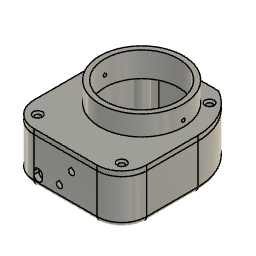
Microscope illuminator (Autodesk Fusion 360 design; units mm, degrees)
Autodesk Fusion 360 part; units mm, degrees
sketch "Sketch1" plane through (0, 0, 0) normal (0, 0, 1) x (1, 0, 0)
  circle A0 centre (0, 0) radius 25.2
  line L0 (-34, 0) -> (0, 0) construction
  line L1 (34, 0) -> (0, 0) construction
  line L2 (-10, 21) -> (10, 21) construction
  line L3 (10, 21) -> (10, -39) construction
  line L4 (10, -39) -> (-10, -39) construction
  line L5 (-10, -39) -> (-10, 21) construction
  line L6 (0, -39) -> (0, 0) construction
  circle A1 centre (0, 0) radius 5 construction
  arc A2 (34, 0) -> (-34, 0) centre (0, 0) ccw
  line L7 (-34, 0) -> (-34, -46)
  line L8 (34, 0) -> (34, -46)
  line L9 (34, -46) -> (-34, -46)
  circle A3 centre (0, 0) radius 22.2
  line L10 (16.9041, 29.5) -> (-16.9041, 29.5)
  line L11 (0, 0) -> (0, 34) construction
  dimension "d3" = 50.4
  dimension "d4" = 68
  dimension "d5" = 60
  dimension "d6" = 20
  dimension "d7" = 39
  dimension "d8" = 10
  dimension "d9" = 3
  dimension "d11" = 46
  dimension "d65" = 4.5
  constraint concentric A0 A2
  constraint coincident A0.centre L0.end
  constraint horizontal L0
  constraint horizontal L2
  constraint vertical L3
  constraint horizontal L4
  constraint vertical L5
  constraint midpoint L4 L6.start
  constraint perpendicular L4 L6
  constraint tangent A2 L7
  constraint tangent A2 L8
  constraint perpendicular L1 L8
  constraint horizontal L9
  constraint concentric A2 A3
  constraint perpendicular L8 L9
  constraint coincident A2 L10.start
  constraint coincident A2 L10.end
  constraint parallel L1 L10
  constraint midpoint A2 L11.end
  measures "d3" diameter of A0
  measures "d4" diameter of A2
  measures "d5" distance of L2.start L4.end
  measures "d6" distance of L2.start L2.end
  measures "d7" distance of L6.start A0.centre
  measures "d8" diameter of A1
  measures "d9" distance of A0 A3
  measures "d11" distance of L0.start L7.end
  measures "d65" distance of L10 L11.end
extrude "Extrude1" add sketch "Sketch1" along normal blind 15 contours A0 makes body 1
extrude "Extrude2" add sketch "Sketch1" along normal blind 3 contours A2 L7 L8 L9 L10 bodies 1
sketch "Sketch Mounting Ring Holes" plane through (0, 0, 0) normal (1, 0, 0) x (0, 1, 0)
  line L0 (0, 15) -> (0, 3) construction
  circle A0 centre (0, 6.5) radius 1
  point P0 (0, 3)
  point P1 (0, 15)
  dimension "d16" = 2
  dimension "d130" = 3.5
  constraint coincident P1 L0.start
  constraint coincident P0 L0.end
  measures "d16" diameter of A0
  measures "d130" distance of P0 A0.centre
extrude "Extrude3" cut sketch "Sketch Mounting Ring Holes" along normal through all and the other way through all bodies 1
fillet "Fillet1" radius 15 2 edges at (-34, -46, 1.5) (34, -46, 1.5) on bodies 1
sketch "Sketch Body Profile" plane through (0, 0, 0) normal (0, 0, 1) x (1, 0, 0)
  arc A0 (19, -46) -> (34, -31) centre (19, -31) ccw
  line L0 (19, -46) -> (-19, -46)
  arc A1 (-34, -31) -> (-19, -46) centre (-19, -31) ccw
  line L1 (-34, -31) -> (-34, 0)
  arc A2 (-16.9041, 29.5) -> (-34, 0) centre (0, 0) ccw
  line L2 (34, 0) -> (34, -31)
  circle A3 centre (0, 0) radius 22.2
  line L3 (-16.9041, 29.5) -> (16.9041, 29.5)
  arc A4 (34, 0) -> (16.9041, 29.5) centre (0, 0) ccw
extrude "Extrude4" add sketch "Sketch Body Profile" against normal blind 27 separate body contours A0 L0 A1 L1 A2 L2 L3 A4 | A3 makes body 2
fillet "Fillet2" radius 3 8 edges at (29.6066, -41.6066, -27) (0, -46, -27) (-29.6066, -41.6066, -27) (-34, -15.5, -27) (-29.4172, 17.0479, -27) (34, -15.5, -27) (29.4172, 17.0479, -27) (0, 29.5, -27) on bodies 2
shell "Shell1" thickness 3 removed faces 1 at (6.3333, -15.3333, 0) on bodies 2
sketch "Sketch Lamp Base Mounting Bosses" plane through (0, -43, 0) normal (0, -1, 0) x (1, 0, 0)
  line L0 (-19, -27) -> (19, -27)
  line L1 (19, -27) -> (19, 0)
  line L2 (19, 0) -> (-19, 0)
  line L3 (-19, 0) -> (-19, -27)
  line L4 (0, 0) -> (0, -27) construction
  circle A0 centre (0, -13.5) radius 6.375 construction
  line L5 (0, -13.5) -> (3.6565, -8.2779) construction
  circle A1 centre (3.6565, -8.2779) radius 1.75
  line L6 (3.6565, -8.2779) -> (-3.6565, -18.7221) construction
  circle A2 centre (-3.6565, -18.7221) radius 1.75
  circle A3 centre (-3.6565, -18.7221) radius 3.75
  circle A4 centre (3.6565, -8.2779) radius 3.75
  line L7 (3.6565, -8.2779) -> (3.6565, -6.5279) construction
  line L8 (3.6565, -6.5279) -> (3.6565, -6.0279) construction
  line L9 (3.6565, -6.0279) -> (4.7565, -6.9168)
  line L10 (3.6565, -6.0279) -> (2.5566, -6.9168)
  line L11 (-3.6565, -18.7221) -> (-3.6565, -16.9721) construction
  line L12 (-3.6565, -16.9721) -> (-3.6565, -16.4721) construction
  line L13 (-3.6565, -16.4721) -> (-2.5566, -17.361)
  line L14 (-3.6565, -16.4721) -> (-4.7565, -17.361)
  line L15 (3.1565, -11.9944) -> (4.1565, -11.9944)
  line L16 (-4.1565, -22.4386) -> (-3.1565, -22.4386)
  line L17 (19, -24) -> (-19, -24)
  line L18 (-19, -24) -> (-19, 0)
  line L19 (-19, 0) -> (19, 0)
  line L20 (19, 0) -> (19, -24)
  dimension "d26" = 35
  dimension "d27" = 3.5
  dimension "d28" = 3.5
  dimension "d31" = 2
  dimension "d32" = 2
  dimension "d66" = 12.75
  dimension "d67" = 0.5
  dimension "d68" = 0.5
  dimension "d69" = 1
  dimension "d70" = 1
  constraint coincident L4.start origin
  constraint midpoint L0 L4.end
  constraint midpoint L4 A0.centre
  constraint coincident A0.centre L5.start
  constraint coincident A0 L5.end
  constraint coincident L5.end A1.centre
  constraint coincident A0 L6.end
  constraint parallel L5 L6
  constraint coincident L6.end A2.centre
  constraint concentric A2 A3
  constraint coincident A1 L7.end
  constraint vertical L7
  constraint parallel L7 L8
  constraint coincident A1 L9.end
  constraint tangent A1 L9
  constraint coincident A1 L10.end
  constraint tangent A1 L10
  constraint coincident A2 L11.end
  constraint vertical L11
  constraint parallel L11 L12
  constraint coincident A2 L13.end
  constraint tangent A2 L13
  constraint coincident A2 L14.end
  constraint tangent A2 L14
  constraint coincident A4 L15.start
  constraint coincident A4 L15.end
  constraint horizontal L15
  constraint coincident A3 L16.start
  constraint coincident A3 L16.end
  constraint horizontal L16
  measures "d26" angle of L4 L5
  measures "d27" diameter of A1
  measures "d28" diameter of A2
  measures "d31" distance of A1 A4
  measures "d32" distance of A2 A3
  measures "d66" distance of L5.end L6.end
  measures "d67" distance of L7.end L8.end
  measures "d68" distance of L11.end L12.end
  measures "d69" distance of L15.start L15.end
  measures "d70" horizontal distance of L16.start L16.end
extrude "Extrude5" add sketch "Sketch Lamp Base Mounting Bosses" against normal blind 3 contours A3 L16 | A4 L15 picked at (-2.8156, -16.3619) picked at (4.4975, -5.9177) bodies 2
extrude "Extrude6" cut sketch "Sketch Lamp Base Mounting Bosses" along normal up to surface (3 mm away) contours A1 | A1 L9 L10 | A2 | A2 L13 L14 bodies 2
box "BoxPrimitive1" add length 3 width 1 height 3 placed x (0, -1, 0) y (-1, 0, 0) z (0, 0, -1) at (4.1565, -40, -11.9944) bodies 2
box "BoxPrimitive2" add length 3 width 1 height 3 placed x (0, -1, 0) y (-1, 0, 0) z (0, 0, -1) at (-3.1565, -40, -22.4386) bodies 2
chamfer "Chamfer2" distance 3 angle 45 1 edges at (3.6565, -40, -14.9944) on bodies 2
sketch "Sketch Screw Bosses in Base" plane through (0, 0, -24) normal (0, 0, 1) x (-1, 0, 0)
  line L0 (-20, 0) -> (-2.5, 0)
  line L1 (0, 0) -> (0, 23.7257) construction
  line L2 (0, 0) -> (-24.0416, -24.0416) construction
  circle A0 centre (-20.5061, -20.5061) radius 4
  arc A1 (16.9041, -29.5) -> (34, 0) centre (0, 0) ccw
  line L3 (-22.5355, 34.5355) -> (-29.6066, 41.6066) construction
  line L4 (-19, 43) -> (19, 43)
  arc A2 (-19, 46) -> (-34, 31) centre (-19, 31) ccw
  circle A3 centre (-25.364, 37.364) radius 4
  circle A4 centre (-20.5061, -20.5061) radius 1.15
  circle A5 centre (-25.364, 37.364) radius 1.15
  circle A6 centre (20.5061, -20.5061) radius 4
  circle A7 centre (20.5061, -20.5061) radius 1.15
  circle A8 centre (25.364, 37.364) radius 4
  circle A9 centre (25.364, 37.364) radius 1.15
  line L5 (31, 0) -> (31, 31)
  arc A10 (31, 31) -> (19, 43) centre (19, 31) ccw
  line L6 (3.1565, 43) -> (-19, 43)
  arc A11 (-19, 43) -> (-31, 31) centre (-19, 31) ccw
  line L7 (-31, 31) -> (-31, 0)
  arc A12 (16.0857, -26.5) -> (31, 0) centre (0, 0) ccw
  arc A13 (-31, 0) -> (-16.0857, -26.5) centre (0, 0) ccw
  line L8 (-16.0857, -26.5) -> (16.0857, -26.5)
  line L9 (4.1565, 43) -> (4.1565, 40)
  line L10 (4.1565, 40) -> (3.1565, 40)
  line L11 (3.1565, 40) -> (3.1565, 43)
  line L12 (19, 43) -> (4.1565, 43)
  dimension "d48" = 45
  dimension "d49" = 8
  dimension "d50" = 5
  dimension "d51" = 45
  dimension "d52" = 8
  dimension "d53" = 6
  dimension "d54" = 2.3
  dimension "d56" = 2.3
  constraint perpendicular L0 L1
  constraint coincident L1.start L2.start
  constraint coincident L2 A0.centre
  constraint coincident L2.end A1
  constraint midpoint L3.end A2
  constraint coincident L3 A3.centre
  constraint concentric A0 A4
  constraint concentric A3 A5
  constraint symmetric L1 A0 A6
  constraint symmetric L1 A3 A8
  constraint symmetric L1 A4 A7
  constraint symmetric L1 A5 A9
  measures "d48" angle of L0 L2
  measures "d49" diameter of A0
  measures "d50" distance of L2.end A0.centre
  measures "d51" angle of L3 L4
  measures "d52" diameter of A3
  measures "d53" distance of L3.end A3.centre
  measures "d54" diameter of A4
  measures "d56" diameter of A5
extrude "Extrude9" add sketch "Sketch Screw Bosses in Base" along normal up to surface (24 mm away) contours A0 A13 | A0 A13 | A3 A11 | A3 A11 | A6 A12 | A6 A12 | A8 A10 | A8 A10 bodies 2
sketch "Sketch Lid Mounting Hole Location" plane through (0, 0, 3) normal (0, 0, 1) x (-1, 0, 0)
  arc A0 (-19, 46) -> (-34, 31) centre (-19, 31) ccw
  line L0 (-34, 31) -> (-34, 0)
  arc A1 (-34, 0) -> (-16.9041, -29.5) centre (0, 0) ccw
  line L1 (34, 0) -> (34, 31)
  arc A2 (34, 31) -> (19, 46) centre (19, 31) ccw
  line L2 (19, 46) -> (-19, 46)
  circle A3 centre (0, 0) radius 25.2
  line L3 (-16.9041, -29.5) -> (16.9041, -29.5)
  arc A4 (16.9041, -29.5) -> (34, 0) centre (0, 0) ccw
  point P0 (25.364, 37.364)
  point P1 (-25.364, 37.364)
  point P2 (20.5061, -20.5061)
  point P3 (-20.5061, -20.5061)
hole "Hole1" at (-25.364, -37.364, 3) at (25.364, -37.364, 3) at (-20.5061, 20.5061, 3) at (20.5061, 20.5061, 3) direction (0, 0, -1) diameter 3.3 depth 4 tip angle 118 countersink diameter 5.5 countersink angle 90 bodies 1
sketch "Sketch Zip Tie Loop" plane through (-31, 0, 0) normal (1, 0, 0) x (0, 1, 0)
  line L0 (0, -24) -> (0, 0)
  line L1 (0, 0) -> (-31, 0)
  line L2 (-31, 0) -> (-31, -24)
  line L3 (-31, -24) -> (0, -24)
  line L4 (-43, -22.4386) -> (-43, -24)
  line L5 (-43, -24) -> (-43, 0)
  line L6 (-43, 0) -> (-43, -24)
  line L7 (-43, -24) -> (-43, -22.4386)
  line L8 (-43, -14.9721) -> (-43, -22.4386)
  line L9 (-43, -14.9944) -> (-43, -11.9944)
  line L10 (-43, -4.5279) -> (-43, -11.9944)
  line L11 (-43, -11.9944) -> (-43, -14.9944)
  line L12 (-24, -24) -> (-24, -16)
  line L13 (-24, -16) -> (-14, -16)
  line L14 (-14, -16) -> (-14, -24)
  line L15 (-43, 0) -> (-43, -24)
  line L16 (-24, -24) -> (-14, -24)
  point P0 (-43, -24)
  point P1 (-43, -24)
  point P2 (-43, -24)
  dimension "d111" = 8
  dimension "d112" = 10
  dimension "d114" = 19
  constraint coincident L3 L12.start
  constraint perpendicular L3 L12
  constraint perpendicular L12 L13
  constraint coincident L3 L14.end
  constraint perpendicular L3 L14
  measures "d111" distance of L12.start L12.end
  measures "d112" distance of L12.end L13.end
  measures "d114" distance of L9.start L12
extrude "Extrude14" add sketch "Sketch Zip Tie Loop" along normal blind 6 contours L3 L12 L13 L14 L16 bodies 2
sketch "Sketch Zip Tie Loop top" plane through (0, 0, -16) normal (0, 0, 1) x (-1, 0, 0)
  line L0 (31, 14) -> (31, 24)
  line L1 (31, 24) -> (25, 24)
  line L2 (25, 24) -> (25, 14)
  line L3 (25, 14) -> (31, 14)
  line L4 (25, 19) -> (31, 19) construction
  line L5 (31, 21.5) -> (27, 21.5)
  line L6 (31, 16.5) -> (27, 16.5)
  line L7 (27, 21.5) -> (27, 16.5)
  line L8 (31, 24) -> (31, 14)
  dimension "d118" = 5
  dimension "d119" = 4
  constraint midpoint L2 L4.start
  constraint midpoint L0 L4.end
  constraint coincident L0 L5.start
  constraint perpendicular L0 L5
  constraint symmetric L4 L5.start L6.start
  constraint symmetric L4 L5.end L6.end
  measures "d118" distance of L5.end L6.end
  measures "d119" distance of L7 L8
extrude "Extrude15" cut sketch "Sketch Zip Tie Loop top" against normal up to surface (8 mm away) contours L0 L5 L6 L7 L8 bodies 2
sketch "Sketch19" plane through (-25, 0, 0) normal (1, 0, 0) x (0, 1, 0)
  line L0 (-24, -16) -> (-24, -24)
  line L1 (-24, -24) -> (-14, -24)
  line L2 (-14, -24) -> (-14, -16)
  line L3 (-14, -16) -> (-24, -16)
  line L4 (-24, -24) -> (-24, -16)
  line L5 (-24, -16) -> (-21.5, -16)
  line L6 (-21.5, -16) -> (-21.5, -24)
  line L7 (-21.5, -24) -> (-16.5, -24)
  line L8 (-16.5, -24) -> (-16.5, -16)
  line L9 (-16.5, -16) -> (-14, -16)
  line L10 (-14, -16) -> (-14, -24)
  line L11 (-14, -24) -> (0, -24)
  line L12 (0, -24) -> (0, 0)
  line L13 (0, 0) -> (-31, 0)
  line L14 (-31, 0) -> (-31, -24)
  line L15 (-31, -24) -> (-24, -24)
  line L16 (-16.5, -19) -> (-21.5, -19)
  line L17 (-21.5, -19) -> (-21.5, -24)
  line L18 (-16.5, -24) -> (-16.5, -19)
  dimension "d124" = 3
  constraint coincident L8 L16.start
  constraint coincident L6 L16.end
  constraint perpendicular L6 L16
  constraint coincident L6.end L7.start
  constraint perpendicular L7 L17
  constraint coincident L7.end L8.start
  constraint perpendicular L7 L18
  measures "d124" distance of L3 L16
extrude "Extrude16" cut sketch "Sketch19" against normal up to surface (6 mm away) contours L1 L6 L7 L8 L16 L17 L18 bodies 2
fillet "Fillet3" radius 1 1 edges at (-31, -19, -24) on bodies 2
chamfer "Chamfer6" distance 1 angle 45 2 edges at (-26, -21.5, -19) (-26, -16.5, -19) on bodies 2
sketch "Sketch Lamp Cord Hole" plane through (0, -43, 0) normal (0, -1, 0) x (1, 0, 0)
  line L0 (-4.1565, -22.4386) -> (-4.1565, -24)
  line L1 (-4.1565, -24) -> (-19, -24)
  line L2 (-19, -24) -> (-19, 0)
  line L3 (-19, 0) -> (19, 0)
  line L4 (19, 0) -> (19, -24)
  line L5 (19, -24) -> (-3.1565, -24)
  line L6 (-3.1565, -24) -> (-3.1565, -22.4386)
  arc A0 (-3.1565, -22.4386) -> (-4.1565, -22.4386) centre (-3.6565, -18.7221) ccw
  line L7 (4.1565, -14.9944) -> (4.1565, -11.9944)
  arc A1 (4.1565, -11.9944) -> (3.1565, -11.9944) centre (3.6565, -8.2779) ccw
  line L8 (3.1565, -11.9944) -> (3.1565, -14.9944)
  line L9 (3.1565, -14.9944) -> (4.1565, -14.9944)
  line L10 (-19, -19) -> (-19, -21)
  arc A2 (-19, -21) -> (-14, -21) centre (-16.5, -21) ccw
  line L11 (-14, -21) -> (-14, -19)
  arc A3 (-14, -19) -> (-19, -19) centre (-16.5, -19) ccw
  line L12 (-16.5, -19) -> (-16.5, -21) construction
  line L13 (-16.5, -19) -> (-16.5, -16.5) construction
  line L14 (-16.5, -21) -> (-16.5, -23.5) construction
  line L15 (-16.5, -20) -> (-19, -12) construction
  line L16 (19, -24) -> (-19, -24) construction
  dimension "d97" = 5
  dimension "d98" = 7
  dimension "d99" = 2.5
  dimension "d100" = 0.5
  constraint tangent L10 A2
  constraint tangent A2 L11
  constraint parallel L10 L11
  constraint tangent L11 A3
  constraint tangent L10 A3
  constraint perpendicular L3 L12
  constraint coincident A3.centre L12.start
  constraint midpoint A3 L13.end
  constraint coincident A2.centre L12.end
  constraint midpoint A2 L14.end
  constraint midpoint L12 L15.start
  constraint midpoint L2 L15.end
  measures "d97" distance of L10 L11
  measures "d98" distance of L13.end L14.end
  measures "d99" horizontal distance of L15.start L15.end
  measures "d100" distance of L14.end L16
extrude "Extrude12" cut sketch "Sketch Lamp Cord Hole" along normal up to surface (3 mm away) contours L2 L10 A2 L11 A3 bodies 2
sketch "Sketch LED Only text" plane through (0, 0, -24) normal (0, 0, 1) x (-1, 0, 0)
  line L0 (31, 24) -> (31, 31)
  arc A0 (31, 31) -> (29.353, 37.0676) centre (19, 31) ccw
  arc A1 (25.0676, 41.353) -> (29.353, 37.0676) centre (25.364, 37.364) ccw
  arc A2 (25.0676, 41.353) -> (19, 43) centre (19, 31) ccw
  line L1 (19, 43) -> (4.1565, 43)
  line L2 (4.1565, 43) -> (4.1565, 40)
  line L3 (4.1565, 40) -> (3.1565, 40)
  line L4 (3.1565, 40) -> (3.1565, 43)
  line L5 (3.1565, 43) -> (-19, 43)
  arc A3 (-19, 43) -> (-25.0676, 41.353) centre (-19, 31) ccw
  arc A4 (-29.353, 37.0676) -> (-25.0676, 41.353) centre (-25.364, 37.364) ccw
  arc A5 (-29.353, 37.0676) -> (-31, 31) centre (-19, 31) ccw
  line L6 (-31, 31) -> (-31, 0)
  arc A6 (-31, 0) -> (-24.3023, -19.2457) centre (0, 0) ccw
  arc A7 (-19.2457, -24.3023) -> (-24.3023, -19.2457) centre (-20.5061, -20.5061) ccw
  arc A8 (-19.2457, -24.3023) -> (-16.0857, -26.5) centre (0, 0) ccw
  line L7 (-16.0857, -26.5) -> (16.0857, -26.5)
  arc A9 (16.0857, -26.5) -> (19.2457, -24.3023) centre (0, 0) ccw
  arc A10 (24.3023, -19.2457) -> (19.2457, -24.3023) centre (20.5061, -20.5061) ccw
  arc A11 (24.3023, -19.2457) -> (31, 0) centre (0, 0) ccw
  line L8 (-24.3023, -19.2457) -> (-24.3023, 33.5074) construction
  line L9 (30, 16.5) -> (30, 21.5)
  line L10 (30, 21.5) -> (25, 21.5)
  line L11 (25, 21.5) -> (25, 24)
  line L12 (25, 24) -> (31, 24)
  line L13 (31, 0) -> (31, 14)
  line L14 (31, 14) -> (25, 14)
  line L15 (25, 14) -> (25, 16.5)
  line L16 (25, 16.5) -> (30, 16.5)
  dimension "d104" = 5
  text T0 "LED ONLY" font "Arial" height 5 align centre spacing 1 along the path L8 letters at x, y, angle (-25.6257, -10.144, 90) (-25.6257, -6.2593, 90) (-25.6257, -1.6004, 90) (-25.6257, 3.444, 90) (-25.6257, 5.3846, 90) (-25.6257, 10.8178, 90) (-25.6257, 15.8621, 90) (-25.6257, 19.7468, 90)
  constraint perpendicular L7 L8
  constraint coincident A6.end A7.end
  constraint coincident A4 L8.end
extrude "Extrude13" cut sketch "Sketch LED Only text" against normal blind 0.5 text T0 bodies 2
equation "d28 = d27"
equation "d31 = d32"
equation "d52 = d49"
named bodies: "Microscope Illuminator Lid", "Microscope Illuminator Base"
